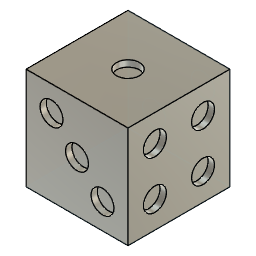
2nd project (Autodesk Fusion 360 design; units mm, degrees)
part number: 2025-07-18-02-54-26-214
part number: 2025-07-18-02-54-51-672
Autodesk Fusion 360 part; units mm, degrees
note: some values were not read from the file. Set by a fixed rule: which sketch regions a step uses.
sketch "Sketch1" plane through (0, 0, 0) normal (0, 0, 1) x (1, 0, 0) in component "Component"
  line L0 (50.8, -50.8) -> (-50.8, -50.8)
  line L1 (-50.8, -50.8) -> (-50.8, 50.8)
  line L2 (-50.8, 50.8) -> (50.8, 50.8)
  line L3 (50.8, 50.8) -> (50.8, -50.8)
  line L4 (50.8, -50.8) -> (-50.8, 50.8) construction
  line L5 (-50.8, -50.8) -> (50.8, 50.8) construction
  dimension "d1" = 101.6
  dimension "d2" = 101.6
  constraint horizontal L0
  constraint perpendicular L0 L1
  constraint parallel L0 L2
  constraint parallel L1 L3
  constraint coincident L4 origin
  constraint coincident L5 origin
  measures "d1" distance of L1.end L2.end
  measures "d2" distance of L0.end L1.end
extrude "Extrude1" add sketch "Sketch1" along normal mid plane 101.6 in component "Component"
sketch "Sketch2" plane through (0, 0, 50.8) normal (0, 0, 1) x (-1, 0, 0) in component "Component"
  line L0 (-50.8, -50.8) -> (50.8, -50.8)
  line L1 (50.8, -50.8) -> (50.8, 50.8)
  line L2 (50.8, 50.8) -> (-50.8, 50.8)
  line L3 (-50.8, 50.8) -> (-50.8, -50.8)
  circle A0 centre (0, 0) radius 11.43
  dimension "d5" = 22.86
  constraint coincident A0.centre origin
  measures "d5" diameter of A0
extrude "Extrude2" cut sketch "Sketch2" against normal blind 6.35 contours A0 in component "Component"
sketch "Sketch3" plane through (0, -50.8, 0) normal (0, -1, 0) x (1, 0, 0) in component "Component"
  line L0 (50.8, -50.8) -> (50.8, 50.8)
  line L1 (50.8, 50.8) -> (-50.8, 50.8)
  line L2 (-50.8, 50.8) -> (-50.8, -50.8)
  line L3 (-50.8, -50.8) -> (50.8, -50.8)
  circle A0 centre (0, 0) radius 11.43
  line L4 (-50.8, 50.8) -> (0, 0)
  line L5 (0, 0) -> (50.8, -50.8)
  circle A1 centre (-25.4, 25.4) radius 11.43
  circle A2 centre (25.4, -25.4) radius 11.43
  dimension "d8" = 22.86
  dimension "d9" = 22.86
  dimension "d10" = 22.86
  constraint coincident A0.centre L4.end
  constraint coincident L1.end L2.start
  constraint coincident L0.start L3.end
  constraint midpoint L4 A1.centre
  constraint midpoint L5 A2.centre
  measures "d8" diameter of A0
  measures "d9" diameter of A1
  measures "d10" diameter of A2
extrude "Extrude3" cut sketch "Sketch3" against normal blind 6.35 contours L5 A2 | L5 A2 | L4 A1 | L4 A1 | A0 L4 L5 | A0 L4 L5 in component "Component"
sketch "Sketch4" plane through (50.8, 0, 0) normal (1, 0, 0) x (0, 1, 0) in component "Component"
  line L0 (50.8, -50.8) -> (50.8, 50.8)
  line L1 (50.8, 50.8) -> (-50.8, 50.8)
  line L2 (-50.8, 50.8) -> (-50.8, -50.8)
  line L3 (-50.8, -50.8) -> (50.8, -50.8)
  line L4 (-50.8, 50.8) -> (50.8, -50.8)
  line L5 (-50.8, -50.8) -> (50.8, 50.8) construction
  circle A0 centre (-23.9624, 23.9624) radius 11.43
  circle A1 centre (23.9624, 23.9624) radius 11.43
  circle A2 centre (-23.9624, -23.9624) radius 11.43
  circle A3 centre (23.9624, -23.9624) radius 11.43
  dimension "d13" = 22.86
  constraint coincident L1.end L2.start
  constraint coincident L0.start L3.end
  constraint coincident L2.end L3.start
  constraint coincident L0.end L1.start
  constraint coincident L4 A0.centre
  constraint coincident L5 A1.centre
  constraint equal A0 A1
  constraint coincident L5 A2.centre
  constraint coincident L4 A3.centre
  constraint equal A1 A3
  constraint equal A1 A2
  measures "d13" diameter of A1
extrude "Extrude4" cut sketch "Sketch4" against normal blind 6.35 contours L4 A3 | L4 A3 | L4 A0 | L4 A0 | A1 | A2 in component "Component"
sketch "Sketch5" plane through (0, 50.8, 0) normal (0, 1, 0) x (-1, 0, 0) in component "Component"
  line L0 (50.8, -50.8) -> (50.8, 50.8)
  line L1 (50.8, 50.8) -> (-50.8, 50.8)
  line L2 (-50.8, 50.8) -> (-50.8, -50.8)
  line L3 (-50.8, -50.8) -> (50.8, -50.8)
  line L4 (-50.8, 50.8) -> (50.8, -50.8)
  circle A0 centre (24.6983, -24.6983) radius 11.43
  circle A1 centre (-23.7784, 23.7784) radius 11.43
  dimension "d16" = 22.86
  constraint coincident L1.end L2.start
  constraint coincident L0.start L3.end
  constraint coincident L4 A0.centre
  constraint coincident L4 A1.centre
  constraint equal A0 A1
  measures "d16" diameter of A0
extrude "Extrude5" cut sketch "Sketch5" against normal blind 6.35 contours L4 A0 | L4 A0 | L4 A1 | L4 A1 in component "Component"
sketch "Sketch6" plane through (-50.8, 0, 0) normal (-1, 0, 0) x (0, -1, 0) in component "Component"
  line L0 (50.8, -50.8) -> (50.8, 50.8)
  line L1 (50.8, 50.8) -> (-50.8, 50.8)
  line L2 (-50.8, 50.8) -> (-50.8, -50.8)
  line L3 (-50.8, -50.8) -> (50.8, -50.8)
  line L4 (-50.8, 50.8) -> (50.8, -50.8)
  line L5 (-50.8, -50.8) -> (50.8, 50.8)
  circle A0 centre (0, 0) radius 12.7
  circle A1 centre (-24.3304, 24.3304) radius 12.7
  circle A2 centre (24.3304, 24.3304) radius 12.7
  circle A3 centre (-24.3304, -24.3304) radius 12.7
  circle A4 centre (24.3304, -24.3304) radius 12.7
  dimension "d19" = 25.4
  constraint coincident L1.end L2.start
  constraint coincident L0.start L3.end
  constraint coincident L2.end L3.start
  constraint coincident L0.end L1.start
  constraint coincident A0.centre origin
  constraint coincident L4 A1.centre
  constraint coincident L5 A2.centre
  constraint coincident L5 A3.centre
  constraint coincident L4 A4.centre
  constraint equal A0 A2
  constraint equal A0 A1
  constraint equal A0 A3
  constraint equal A0 A4
  measures "d19" diameter of A0
extrude "Extrude6" cut sketch "Sketch6" against normal blind 6.35 contours L4 A4 | L4 A4 | L5 A2 | L5 A2 | L5 A3 | L5 A3 | L4 A1 | L4 A1 | L4 L5 A0 | L4 L5 A0 | L4 L5 A0 | L4 L5 A0 in component "Component"
sketch "Sketch7" plane through (0, 0, -50.8) normal (0, 0, -1) x (1, 0, 0) in component "Component"
  line L0 (-50.8, -50.8) -> (50.8, -50.8)
  line L1 (50.8, -50.8) -> (50.8, 50.8)
  line L2 (50.8, 50.8) -> (-50.8, 50.8)
  line L3 (-50.8, 50.8) -> (-50.8, -50.8)
sketch "Sketch8" plane through (0, 50.8, 0) normal (0, 1, 0) x (-1, 0, 0) in component "Component"
  circle A0 centre (24.6983, -24.6983) radius 11.43
  circle A1 centre (-23.7784, 23.7784) radius 11.43
  line L0 (50.8, -50.8) -> (50.8, 50.8)
  line L1 (50.8, 50.8) -> (-50.8, 50.8)
  line L2 (-50.8, 50.8) -> (-50.8, -50.8)
  line L3 (-50.8, -50.8) -> (50.8, -50.8)
sketch "Sketch10" plane through (0, 0, -50.8) normal (0, 0, -1) x (1, 0, 0) in component "Component"
component "Component" placed x (1, 0, 0) y (0, 1, 0) z (0, 0, 1) at (0, 0, 0)
equation "d1 = dicesize"
equation "d2 = dicesize"
equation "d5 = Divotsize"
equation "d8 = Divotsize"
equation "d9 = Divotsize"
equation "d10 = Divotsize"
equation "d13 = Divotsize"
equation "d16 = Divotsize"
equation "dicesize = 4 in"
equation "Divotsize = 0.9 in"
equation "diceDepth = 0.25 in"
